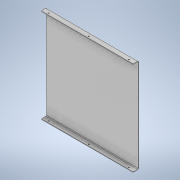
# Autodesk Inventor part: Platform top
Saved by Autodesk Inventor 2020 (Build 240168000, 168)
## iProperties
Created: 2022-07-05
Part Number: Platform top
Material: Generic
Document SubType Name: Sheet Metal
Designer: karimi2
Density: 1 g/cm^3
Sheet Metal Rule: Default_mm
Appearance: Aluminum - Polished
Author: karimi2
Autodesk Inventor part; units mm, degrees
ref_plane "YZ Plane" through (0, 0, 0) normal (1, 0, 0) x (0, 1, 0)
ref_plane "XZ Plane" through (0, 0, 0) normal (0, 1, 0) x (-1, 0, 0)
ref_plane "XY Plane" through (0, 0, 0) normal (0, 0, 1) x (1, 0, 0)
sketch "Sketch1" plane through (0, 0, 0) normal (0, 0, 1) x (1, 0, 0)
  line L0 (160, -180) -> (-160, -180)
  line L1 (-160, -180) -> (-160, 180)
  line L2 (-160, 180) -> (160, 180)
  line L3 (160, 180) -> (160, -180)
  circle A0 centre (-140, 174.524) radius 2
  circle A1 centre (0, 174.524) radius 2
  circle A2 centre (140, 174.524) radius 2
  circle A3 centre (-140, -174.524) radius 2
  circle A4 centre (0, -174.524) radius 2
  circle A5 centre (140, -174.524) radius 2
  point P0 (0, 0)
  dimension "d2" = 320
  dimension "d3" = 360
  dimension "d4" = 20
  dimension "d5" = 5.476
  dimension "d6" = 5.476
  dimension "d7" = 20
  dimension "d8" = 4
  dimension "d31" = 180
  dimension "d32" = 160
  measures "d2" distance of L1.end L2.end
  measures "d3" distance of L2.end L0.start
  measures "d4" distance from line of L1 A0.centre
  measures "d5" distance from line of L2 A0.centre
  measures "d6" distance from line of L0 A3.centre
  measures "d7" distance from line of L3 A2.centre
  measures "d8" diameter of A0
  measures "d31" distance from line of point (0, 0) L0
  measures "d32" distance from line of point (0, 0) L3
extrude "Plate1" add sketch "Sketch1" along normal blind 2
sketch "Sketch2" plane through (0, 0, 2) normal (0, 0, 1) x (1, 0, 0)
  line L0 (-160, -180) -> (-160, 180) projected
  line L1 (-160, 160) -> (160, 160)
  line L2 (160, 180) -> (160, -180) projected
  line L3 (-160, 180) -> (160, 180) projected
  point P0 (0, 0)
  dimension "d10" = 20
  constraints: 2 end point, 2 point on line, 1 horizontal
  measures "d10" distance between parallel lines of L3 L1
fold "Fold1" angle 90 bend radius 2 thickness 2 k factor 0.44 line from (-160, 160, 2) to (160, 160, 2) line at bend start moving side (0, 1, 0) folds toward (0, 0, 1)
sketch "Sketch3" plane through (0, 0, 2) normal (0, 0, 1) x (1, 0, 0)
  line L0 (-160, -180) -> (-160, 160) projected
  line L1 (-160, -160) -> (160, -160)
  line L2 (160, 160) -> (160, -180) projected
  line L3 (160, -180) -> (-160, -180) projected
  point P0 (0, 0)
  dimension "d17" = 20
  constraints: 2 end point, 2 point on line, 1 horizontal
  measures "d17" distance between parallel lines of L3 L1
fold "Fold3" angle 90 bend radius 2 thickness 2 k factor 0.44 line from (-160, -160, 2) to (160, -160, 2) line at bend start moving side (0, -1, 0) folds toward (0, 0, 1)
fillet "Fillet1" radius 2 4 edges at (160, 163, 19.4761) (160, -163, 19.4761) (-160, 163, 19.4761) (-160, -163, 19.4761)
equation "\"d9\" = Thickness"
equation "\"d11\" = BendReliefWidth"
equation "\"d12\" = BendReliefDepth"
equation "\"d13\" = MinimumRemnant"
equation "\"d14\" = TransitionRadius"
equation "\"d16\" = BendRadius"
equation "\"d24\" = BendReliefWidth"
equation "\"d25\" = BendReliefDepth"
equation "\"d26\" = MinimumRemnant"
equation "\"d27\" = TransitionRadius"
equation "\"d29\" = BendRadius"
equation "\"BendRadius\" = Thickness"
equation "\"BendReliefWidth\" = Thickness"
equation "\"BendReliefDepth\" = 0.5 * Thickness"
equation "\"CornerReliefSize\" = 4 * Thickness"
equation "\"MinimumRemnant\" = 2 * Thickness"
equation "\"TransitionRadius\" = BendRadius"
equation "\"JacobiRadiusSize\" = BendRadius"
equation "\"GapSize\" = Thickness"
equation "\"Thickness\" = 2"
body "Solid1"
